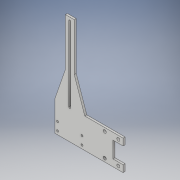
# Autodesk Inventor part: Upper_plate
Saved by Autodesk Inventor 2019 (Build 230136000, 136)
## iProperties
Created: 2018-10-09
Part Number: Upper_plate
Material: Generisch
Document SubType Name: Modeling
Designer: janbe
Density: 1 g/cm^3
Appearance: Vorgabe
Author: janbe
Autodesk Inventor part; units mm, degrees
ref_plane "YZ Plane" through (0, 0, 0) normal (1, 0, 0) x (0, 1, 0)
ref_plane "XZ Plane" through (0, 0, 0) normal (0, 1, 0) x (-1, 0, 0)
ref_plane "XY Plane" through (0, 0, 0) normal (0, 0, 1) x (1, 0, 0)
sketch "Skizze1" plane through (0, 0, 0) normal (0, 0, 1) x (1, 0, 0)
  circle A0 centre (0, 0) radius 2.3
  line L0 (-73.5, 5) -> (27, 5)
  line L1 (27, -39) -> (-73.5, -39)
  line L2 (-73.5, -39) -> (-73.5, 5)
  circle A1 centre (20, 0) radius 2.3
  circle A2 centre (0, -34) radius 2.3
  circle A3 centre (20, -34) radius 2.3
  line L3 (27, -29) -> (12, -29)
  line L4 (12, -29) -> (12, -5)
  line L5 (12, -5) -> (27, -5)
  line L6 (27, 5) -> (27, -5)
  line L7 (27, -29) -> (27, -39)
  dimension "d0" = 4.6
  dimension "d3" = 20
  dimension "d6" = 34
  dimension "d9" = 10
  dimension "d11" = 5
  dimension "d12" = 5
  dimension "d13" = 5
  dimension "d15" = 15
  dimension "d16" = 7
  dimension "d17" = 100.5
  constraints: 16 end point, 4 centre point, 4 parallel, 3 horizontal, 3 perpendicular, 1 coincident, 1 collinear, 1 vertical, 6 other
  measures "d0" diameter of A0
  measures "d3" distance of A0.centre A1.centre
  measures "d6" distance of A0.centre A2.centre
  measures "d9" distance between parallel lines of L0 L5
  measures "d11" distance from line of A1.centre L0
  measures "d12" distance from line of L1 A3.centre
  measures "d13" distance from line of L3 A3.centre
  measures "d15" distance between parallel lines of L6 L4
  measures "d16" distance from line of L6 A1.centre
  measures "d17" distance between parallel lines of L2 L6
extrude "Extrusion1" add sketch "Skizze1" along normal blind 3
sketch "Skizze2" plane through (0, 0, 3) normal (0, 0, 1) x (1, 0, 0)
  circle A0 centre (-69.5, -34) radius 1.5
  circle A1 centre (20, -34) radius 2.3 projected
  circle A2 centre (0, -34) radius 2.3 projected
  circle A3 centre (20, 0) radius 2.3 projected
  circle A4 centre (0, 0) radius 2.3 projected
  line L0 (27, 5) -> (-73.5, 5) projected
  line L1 (-73.5, 5) -> (-73.5, -39) projected
  line L2 (-73.5, -39) -> (27, -39) projected
  line L3 (27, -39) -> (27, -29) projected
  line L4 (27, -29) -> (12, -29) projected
  line L5 (12, -29) -> (12, -5) projected
  line L6 (12, -5) -> (27, -5) projected
  line L7 (27, -5) -> (27, 5) projected
  circle A5 centre (-33.5, -34) radius 1.5
  circle A6 centre (-69.5, -22) radius 1.5
  circle A7 centre (-33.5, -22) radius 1.5
  dimension "d20" = 3
  dimension "d21" = 5
  dimension "d22" = 4
  dimension "d25" = 36
  dimension "d28" = 12
  constraints: 4 centre point, 1 horizontal, 1 vertical, 6 other
  measures "d20" diameter of A0
  measures "d21" distance from line of A0.centre L2
  measures "d22" distance from line of A0.centre L1
  measures "d25" distance of A0.centre A5.centre
  measures "d28" distance of A0.centre A6.centre
extrude "Extrusion2" cut sketch "Skizze2" against normal up to surface (3 mm away) contours A0 | A5 | A6 | A7
sketch "Skizze3" plane through (0, 0, 3) normal (0, 0, 1) x (1, 0, 0)
  circle A0 centre (-69.5, -22) radius 1.5 projected
  circle A1 centre (-33.5, -22) radius 1.5 projected
  circle A2 centre (-33.5, -34) radius 1.5 projected
  circle A3 centre (-69.5, -34) radius 1.5 projected
  circle A4 centre (20, -34) radius 2.3 projected
  circle A5 centre (0, -34) radius 2.3 projected
  circle A6 centre (20, 0) radius 2.3 projected
  circle A7 centre (0, 0) radius 2.3 projected
  line L0 (27, 5) -> (-73.5, 5) projected
  line L1 (-73.5, 5) -> (-73.5, -39) projected
  line L2 (-73.5, -39) -> (27, -39) projected
  line L3 (27, -39) -> (27, -29) projected
  line L4 (27, -29) -> (12, -29) projected
  line L5 (12, -29) -> (12, -5) projected
  line L6 (12, -5) -> (27, -5) projected
  line L7 (27, -5) -> (27, 5) projected
  line L8 (-73.5, 5) -> (-29.5, 5)
  line L9 (-29.5, 5) -> (-29.5, 5.1)
  line L10 (-29.5, 5.1) -> (-73.5, 5.1)
  line L11 (-73.5, 5.1) -> (-73.5, 5)
  line L12 (-53, 5.1) -> (-50, 5.1)
  line L13 (-50, 5.1) -> (-50, 115.1)
  line L14 (-50, 115.1) -> (-53, 115.1)
  line L15 (-53, 115.1) -> (-53, 5.1)
  line L16 (-58, 5.1) -> (-45, 5.1)
  line L17 (-45, 5.1) -> (-45, 120.1)
  line L18 (-45, 120.1) -> (-58, 120.1)
  line L19 (-58, 120.1) -> (-58, 5.1)
  line L20 (-73.5, 5.1) -> (-58, 50.1)
  line L21 (-29.5, 5.1) -> (-45, 50.1)
  dimension "d33" = 44
  dimension "d34" = 0.1
  dimension "d35" = 3
  dimension "d36" = 110
  dimension "d37" = 5
  dimension "d38" = 5
  dimension "d39" = 5
  dimension "d40" = 15.5
  dimension "d41" = 45
  dimension "d42" = 45
  dimension "d46" = 15.5
  dimension "d47" = 16.5
  dimension "d48" = 16.5
  constraints: 28 end point, 6 parallel, 4 point on line, 3 horizontal, 3 perpendicular
  measures "d33" distance of L10.end L9.end
  measures "d34" distance of L10.end L0.end
  measures "d35" distance of L14.end L13.end
  measures "d36" distance of L13.end L12.end
  measures "d37" distance between parallel lines of L18 L14
  measures "d38" distance between parallel lines of L17 L13
  measures "d39" distance between parallel lines of L19 L15
  measures "d40" distance between parallel lines of L19 L1
  measures "d41" distance from line of L10 L20.end
  measures "d42" distance from line of L10 L21.end
  measures "d46" distance between parallel lines of L9 L17
  measures "d47" distance from line of L15 A0.centre
  measures "d48" distance from line of L13 A1.centre
extrude "Extrusion3" add sketch "Skizze3" against normal up to surface (3 mm away) contours L0 L11 L10 L9 | L10 L17 L21 | L20 L19 L10 | L10 L13 L14 L15 L19 L18 L17
sketch "Skizze4" plane through (0, 0, 3) normal (0, 0, 1) x (1, 0, 0)
  line L0 (-53, 5.1) -> (-53, 115.1) projected
  line L1 (-53, 115.1) -> (-50, 115.1) projected
  line L2 (-50, 115.1) -> (-50, 5.1) projected
  line L3 (-50, 5.1) -> (-53, 5.1) projected
  circle A0 centre (-69.5, -22) radius 1.5 projected
  circle A1 centre (-33.5, -22) radius 1.5 projected
  circle A2 centre (-33.5, -34) radius 1.5 projected
  circle A3 centre (-69.5, -34) radius 1.5 projected
  circle A4 centre (20, -34) radius 2.3 projected
  circle A5 centre (0, -34) radius 2.3 projected
  circle A6 centre (20, 0) radius 2.3 projected
  circle A7 centre (0, 0) radius 2.3 projected
  line L4 (27, 5) -> (-29.5, 5) projected
  line L5 (-29.5, 5) -> (-29.5, 5.1) projected
  line L6 (-29.5, 5.1) -> (-45, 50.1) projected
  line L7 (-45, 50.1) -> (-45, 120.1) projected
  line L8 (-45, 120.1) -> (-58, 120.1) projected
  line L9 (-58, 120.1) -> (-58, 50.1) projected
  line L10 (-58, 50.1) -> (-73.5, 5.1) projected
  line L11 (-73.5, 5.1) -> (-73.5, -39) projected
  line L12 (-73.5, -39) -> (27, -39) projected
  line L13 (27, -39) -> (27, -29) projected
  line L14 (27, -29) -> (12, -29) projected
  line L15 (12, -29) -> (12, -5) projected
  line L16 (12, -5) -> (27, -5) projected
  line L17 (27, -5) -> (27, 5) projected
  arc A8 (-50, 115.1) -> (-53, 115.1) centre (-51.5, 115.1) ccw
  line L18 (-50, 5.1) -> (-53, 5.1) projected
  arc A9 (-53, 5.1) -> (-50, 5.1) centre (-51.5, 5.1) ccw
  constraints: 4 point on circle, 3 tangent, 2 centre point
extrude "Extrusion4" cut sketch "Skizze4" against normal up to surface (3 mm away) contours L3 A9 | A8 L1
sketch "Skizze6" plane through (0, 0, 3) normal (0, 0, 1) x (1, 0, 0)
  line L0 (27, 5) -> (-29.5, 5) projected
  line L1 (-29.5, 5) -> (-29.5, 5.1) projected
  line L2 (-29.5, 5.1) -> (-45, 50.1) projected
  line L3 (-45, 50.1) -> (-45, 120.1) projected
  line L4 (-45, 120.1) -> (-58, 120.1) projected
  line L5 (-58, 120.1) -> (-58, 50.1) projected
  line L6 (-58, 50.1) -> (-73.5, 5.1) projected
  line L7 (-73.5, 5.1) -> (-73.5, -39) projected
  line L8 (-73.5, -39) -> (27, -39) projected
  line L9 (27, -39) -> (27, -29) projected
  line L10 (27, -29) -> (12, -29) projected
  line L11 (12, -29) -> (12, -5) projected
  line L12 (12, -5) -> (27, -5) projected
  line L13 (27, -5) -> (27, 5) projected
  circle A0 centre (0, 0) radius 2.3 projected
  circle A1 centre (20, 0) radius 2.3 projected
  circle A2 centre (0, -34) radius 2.3 projected
  circle A3 centre (20, -34) radius 2.3 projected
  circle A4 centre (-69.5, -34) radius 1.5 projected
  circle A5 centre (-33.5, -34) radius 1.5 projected
  circle A6 centre (-33.5, -22) radius 1.5 projected
  circle A7 centre (-69.5, -22) radius 1.5 projected
  arc A8 (-53, 5.1) -> (-50, 5.1) centre (-51.5, 5.1) ccw projected
  line L14 (-53, 5.1) -> (-53, 115.1) projected
  arc A9 (-50, 115.1) -> (-53, 115.1) centre (-51.5, 115.1) ccw projected
  line L15 (-50, 115.1) -> (-50, 5.1) projected
